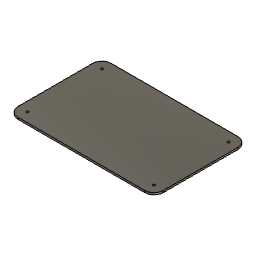
037308-01 Speaker Grille (Autodesk Fusion 360 design; units mm, degrees)
Autodesk Fusion 360 part; units mm, degrees
note: some values were not read from the file. Chosen so that the rebuilt part matches the saved one: a side.
sketch "Sketch1" plane through (0, 0, 0) normal (0, 0, 1) x (1, 0, 0)
  line L0 (86.2521, 63.5) -> (-86.2521, 63.5)
  line L1 (-98.9521, 50.8) -> (-98.9521, -50.8)
  line L2 (-86.2521, -63.5) -> (86.2521, -63.5)
  line L3 (98.9521, -50.8) -> (98.9521, 50.8)
  circle A0 centre (-86.2521, 50.8) radius 1.5875
  circle A1 centre (86.2521, 50.8) radius 1.5875
  circle A2 centre (86.2521, -50.8) radius 1.5875
  circle A3 centre (-86.2521, -50.8) radius 1.5875
  arc A4 (-86.2521, 63.5) -> (-98.9521, 50.8) centre (-86.2521, 50.8) ccw
  arc A5 (98.9521, 50.8) -> (86.2521, 63.5) centre (86.2521, 50.8) ccw
  arc A6 (-98.9521, -50.8) -> (-86.2521, -63.5) centre (-86.2521, -50.8) ccw
  arc A7 (86.2521, -63.5) -> (98.9521, -50.8) centre (86.2521, -50.8) ccw
  line L4 (-98.952, 0) -> (98.952, 0) construction
  point P0 (-98.9521, -63.5)
  point P1 (98.9521, -63.5)
  dimension "d1" = 197.9041
  dimension "d4" = 12.7
  dimension "d5" = 12.7
  dimension "d6" = 12.7
  dimension "d7" = 12.7
  dimension "d8" = 12.7
  dimension "d9" = 12.7
  dimension "d10" = 12.7
  dimension "d11" = 12.7
  dimension "d13" = 3.175
  dimension "d20" = 127
  dimension "d21" = 101.6
  dimension "d22" = 12.7
  dimension "d23" = 172.5041
  constraint horizontal L0
  constraint perpendicular L0 L1
  constraint parallel L0 L2
  constraint parallel L1 L3
  constraint equal A0 A1
  constraint equal A1 A2
  constraint equal A2 A3
  constraint tangent L1 A4
  constraint tangent L0 A4
  constraint tangent L0 A5
  constraint tangent L3 A5
  constraint equal A4 A5
  constraint coincident P0 L1
  constraint coincident P0 L2
  constraint tangent L1 A6
  constraint tangent L2 A6
  constraint coincident P1 L2
  constraint coincident P1 L3
  constraint tangent L2 A7
  constraint tangent L3 A7
  constraint equal A5 A7
  constraint equal A6 A7
  constraint midpoint L1 L4.start
  constraint midpoint L3 L4.end
  constraint midpoint L4 origin
  measures "d1" distance of P0 P1
  measures "d4" distance of L1 A0.centre
  measures "d5" distance of L0 A0.centre
  measures "d6" distance of L0 A1.centre
  measures "d7" distance of L3 A1.centre
  measures "d8" distance of L3 A2.centre
  measures "d9" distance of L2 A2.centre
  measures "d10" distance of L1 A3.centre
  measures "d11" distance of L2 A3.centre
  measures "d13" diameter of A0
  measures "d20" distance of L0 L2
  measures "d21" distance of L1.start L1.end
  measures "d22" radius of A4
  measures "d23" distance of L0.end L0.start
extrude "Face1" add sketch "Sketch1" against normal blind 2.5
equation "MountingHoleOffset = ( 1 / 2 ) * 1 in"
equation "d4 = MountingHoleOffset"
equation "d5 = MountingHoleOffset"
equation "d6 = MountingHoleOffset"
equation "d7 = MountingHoleOffset"
equation "d8 = MountingHoleOffset"
equation "d9 = MountingHoleOffset"
equation "d10 = MountingHoleOffset"
equation "d11 = MountingHoleOffset"
equation "MountingHole = ( 1 / 8 ) * 1 in" comment "Rivet hole"
equation "d13 = MountingHole"
equation "d22 = ( 1 / 2 ) * 1 in"
equation "PerforatedSheetMetalSpacing = ( 1 / 8 ) * 1 in" comment "Spacing of holes in perforated sheet metal"
equation "PerforatedSheetMetalThickness = ( 1 / 16 ) * 1 in"
equation "PerforatedSheetHoleDiameter = ( 1 / 16 ) * 1 in"
